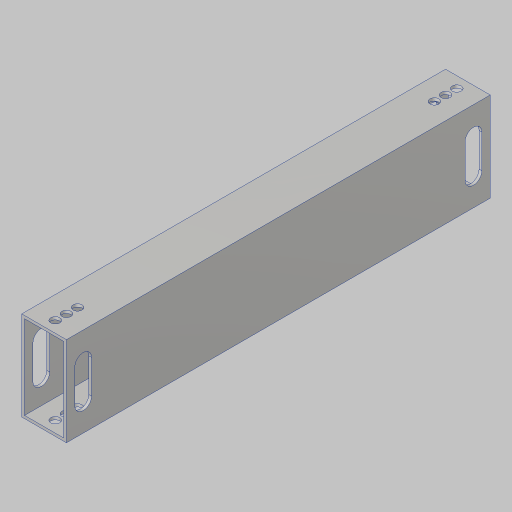
# Autodesk Inventor part: EL2-011
Saved by Autodesk Inventor 2023.5 (Build 275446000, 446)
## iProperties
RuleStatus: InUse
Created: 2025-01-11
Part Number: EL2-011
Material: Aluminum 6061
Document SubType Name: Modeling
Designer: mavericks
Mass: 304.185 g
Surface Area: 718.547 cm^2
Volume: 112.661 cm^3
Density: 2.7 g/cm^3
Appearance: Aluminum - Flat
AfterDocNew0: SHOW
AfterDocOpen0: SHOW
Author: mavericks
Autodesk Inventor part; units mm, degrees
ref_plane "YZ Plane" through (0, 0, 0) normal (1, 0, 0) x (0, 1, 0)
ref_plane "XZ Plane" through (0, 0, 0) normal (0, 1, 0) x (-1, 0, 0)
ref_plane "XY Plane" through (0, 0, 0) normal (0, 0, 1) x (1, 0, 0)
sketch "Sketch1" plane through (0, 0, 0) normal (0, 0, 1) x (1, 0, 0)
  line L0 (-12.7, -25.4) -> (12.7, -25.4)
  line L1 (12.7, -25.4) -> (12.7, 25.4)
  line L2 (12.7, 25.4) -> (-12.7, 25.4)
  line L3 (-12.7, 25.4) -> (-12.7, -25.4)
  line L4 (-12.7, -25.4) -> (12.7, 25.4) construction
  line L5 (12.7, -25.4) -> (-12.7, 25.4) construction
  line L6 (-11.1125, 23.8125) -> (11.1125, 23.8125)
  line L7 (11.1125, 23.8125) -> (11.1125, -23.8125)
  line L8 (11.1125, -23.8125) -> (-11.1125, -23.8125)
  line L9 (-11.1125, -23.8125) -> (-11.1125, 23.8125)
  point P0 (0, 0)
  dimension "width" = 25.4
  dimension "height" = 50.8
  dimension "thickness" = 1.5875
  constraints: 20 end point, 4 parallel, 2 midpoint, 2 perpendicular, 1 horizontal, 3 other
  measures "width" distance of L2.end L1.end
  measures "height" distance of L1.end L0.end
  measures "thickness" distance between parallel lines of L2 L6
extrude "Extrusion1" add sketch "Sketch1" along normal mid plane 241.046
sketch "Sketch3" plane through (-12.7, 25.4, 120.523) normal (0, 1, 0) x (1, 0, 0)
  line L0 (25.4, 0) -> (0, 0) projected
  line L1 (0, 241.046) -> (0, 0) construction
  line L2 (0, 241.046) -> (25.4, 241.046) construction
  point P0 (12.7, 120.523)
  point P1 (12.7, 6.35)
  point P2 (12.7, 12.7)
  point P3 (12.7, 19.05)
  point P4 (12.7, 234.696)
  point P5 (12.7, 228.346)
  point P6 (12.7, 221.996)
  dimension "d18" = 6.35
  dimension "d19" = 6.35
  dimension "d20" = 6.35
  dimension "d21" = 12.7
  dimension "d22" = 6.35
  dimension "d23" = 6.35
  dimension "d24" = 6.35
  constraints: 5 vertical alignment
  measures "d18" distance from line of L0 point (12.7, 6.35)
  measures "d19" distance of point (12.7, 12.7) point (12.7, 6.35)
  measures "d20" distance of point (12.7, 19.05) point (12.7, 12.7)
  measures "d21" distance from line of L1 point (12.7, 6.35)
  measures "d22" distance of point (12.7, 228.346) point (12.7, 221.996)
  measures "d23" distance of point (12.7, 234.696) point (12.7, 228.346)
  measures "d24" distance from line of L2 point (12.7, 234.696)
hole "Hole2" at (0, 25.4, 114.173) at (0, 25.4, 107.823) at (0, 25.4, 101.473) at (0, 25.4, -101.473) at (0, 25.4, -107.823) at (0, 25.4, -114.173) direction (0, -1, 0) diameter 5.1054 end through all clearance for "Flat Head Machine Screw (82)" size "#10" standard "Ansi Unified Screw Threads"
sketch "Sketch4" plane through (12.7, -25.4, 120.523) normal (1, 0, 0) x (0, 0, -1)
  line L0 (9.525, 34.925) -> (9.525, 15.875) construction
  line L1 (4.7625, 34.925) -> (4.7625, 15.875)
  line L2 (14.2875, 15.875) -> (14.2875, 34.925)
  arc A0 (14.2875, 34.925) -> (4.7625, 34.925) centre (9.525, 34.925) ccw
  arc A1 (4.7625, 15.875) -> (14.2875, 15.875) centre (9.525, 15.875) ccw
  line L3 (0, 0) -> (0, 50.8) construction
  line L4 (120.523, 25.4) -> (120.523, 50.8) construction
  line L5 (241.046, 50.8) -> (0, 50.8) construction
  line L6 (231.521, 34.925) -> (231.521, 15.875) construction
  line L7 (236.2835, 34.925) -> (236.2835, 15.875)
  line L8 (226.7585, 15.875) -> (226.7585, 34.925)
  arc A2 (236.2835, 34.925) -> (226.7585, 34.925) centre (231.521, 34.925) ccw
  arc A3 (226.7585, 15.875) -> (236.2835, 15.875) centre (231.521, 15.875) ccw
  point P0 (9.525, 25.4)
  point P1 (231.521, 25.4)
  dimension "d32" = 9.525
  dimension "d33" = 19.05
  dimension "d34" = 9.525
  constraints: 18 end point, 8 point on circle, 7 symmetric about line, 4 centre point, 4 tangent, 2 midpoint, 1 horizontal alignment, 1 parallel, 1 vertical, 2 other
  measures "d32" diameter of A1
  measures "d33" distance of L0.end L0.start
  measures "d34" distance from line of L3 point (9.525, 25.4)
extrude "Extrusion2" cut sketch "Sketch4" against normal through all
equation "\"d20\" = d19"
equation "\"d23\" = d22"
equation "\"d24\" = d23"
body "Solid1"
